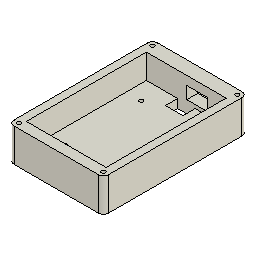
Peekabot 3d design part 1 v1 v21 (Autodesk Fusion 360 design; units mm, degrees)
Autodesk Fusion 360 part; units mm, degrees
sketch "Sketch1" plane through (0, 0, 0) normal (0, 0, 1) x (1, 0, 0)
  line L0 (17.25, -24.75) -> (-17.25, -24.75)
  line L1 (-17.25, -24.75) -> (-17.25, 24.75)
  line L2 (-17.25, 24.75) -> (17.25, 24.75)
  line L3 (17.25, 24.75) -> (17.25, -24.75)
  line L4 (17.25, -24.75) -> (-17.25, 24.75) construction
  line L5 (-17.25, -24.75) -> (17.25, 24.75) construction
  line L6 (-17.25, -24.75) -> (-14.2497, -21.7497)
  line L7 (-17.25, -24.75) -> (-13.007, -24.75) construction
  circle A0 centre (-14.2497, -21.7497) radius 1.115
  line L8 (17.25, -24.75) -> (13.7498, -21.7499)
  line L9 (17.25, -24.75) -> (21.86, -24.75) construction
  circle A1 centre (13.7498, -21.7499) radius 1.115
  line L10 (17.25, 24.75) -> (13.7498, 21.7499)
  line L11 (17.25, 24.75) -> (21.86, 24.75) construction
  circle A2 centre (13.7498, 21.7499) radius 1.1
  line L12 (-17.25, 24.75) -> (-14.2497, 21.7497)
  line L13 (-17.25, 24.75) -> (-13.007, 24.75) construction
  circle A3 centre (-14.2497, 21.7497) radius 1.115
  circle A4 centre (-14.2497, 21.7497) radius 2
  circle A5 centre (13.7498, 21.7499) radius 2
  circle A6 centre (13.7498, -21.7499) radius 2
  circle A7 centre (-14.2497, -21.7497) radius 2
  line L14 (22.25, 29.75) -> (22.25, -29.75)
  line L15 (22.25, -29.75) -> (-22.25, -29.75)
  line L16 (-22.25, -29.75) -> (-22.25, 29.75)
  line L17 (-22.25, 29.75) -> (22.25, 29.75)
  line L18 (27, -41) -> (-27, -41)
  line L19 (-27, -41) -> (-27, 41)
  line L20 (-27, 41) -> (27, 41)
  line L21 (27, 41) -> (27, -41)
  line L22 (27, -41) -> (-27, 41) construction
  line L23 (-27, -41) -> (27, 41) construction
  dimension "d1" = 34.5
  dimension "d2" = 49.5
  dimension "d3" = 45
  dimension "d4" = 4.243
  dimension "d5" = 2.23
  dimension "d6" = 139.4
  dimension "d7" = 4.61
  dimension "d8" = 2.23
  dimension "d9" = 139.4
  dimension "d10" = 4.61
  dimension "d11" = 2.2
  dimension "d12" = 45
  dimension "d13" = 4.243
  dimension "d14" = 2.23
  dimension "d15" = 4
  dimension "d16" = 4
  dimension "d17" = 4
  dimension "d18" = 4
  dimension "d21" = -5
  dimension "d57" = 54
  dimension "d58" = 82
  constraint horizontal L0
  constraint perpendicular L0 L1
  constraint parallel L0 L2
  constraint parallel L1 L3
  constraint coincident L4 origin
  constraint coincident L5 origin
  constraint horizontal L7
  constraint coincident L6.end A0.centre
  constraint horizontal L9
  constraint coincident L8.end A1.centre
  constraint horizontal L11
  constraint coincident L10.end A2.centre
  constraint horizontal L13
  constraint coincident L12.end A3.centre
  constraint concentric A3 A4
  constraint concentric A2 A5
  constraint concentric A1 A6
  constraint concentric A0 A7
  constraint horizontal L18
  constraint perpendicular L18 L19
  constraint parallel L18 L20
  constraint parallel L19 L21
  constraint coincident L22 origin
  constraint coincident L23 origin
  measures "d1" distance of L1.end L2.end
  measures "d2" distance of L0.end L1.end
  measures "d3" angle of L6 L7
  measures "d4" distance of L0.end L6.end
  measures "d5" diameter of A0
  measures "d6" angle of L8 L9
  measures "d7" distance of L0.start L8.end
  measures "d8" diameter of A1
  measures "d9" angle of L10 L11
  measures "d10" distance of L2.end L10.end
  measures "d11" diameter of A2
  measures "d12" angle of L12 L13
  measures "d13" distance of L1.end L12.end
  measures "d14" diameter of A3
  measures "d15" diameter of A4
  measures "d16" diameter of A5
  measures "d17" diameter of A6
  measures "d18" diameter of A7
  measures "d57" distance of L19.end L20.end
  measures "d58" distance of L18.end L19.end
extrude "Extrude1" add sketch "Sketch1" along normal blind 5 contours L0 L1 L2 L3 | A4 | A5 | A6 | A7 makes body 1
extrude "Extrude2" add sketch "Sketch1" along normal blind 5 separate body contours L0 L1 L2 L3 | A4 | A5 | A6 | A7 | L14 L15 L16 L17 makes body 2
extrude "Extrude3" add sketch "Sketch1" along normal blind 19 contours L14 L15 L16 L17 bodies 1 2
extrude "Extrude4" add sketch "Sketch1" against normal blind 5 contours L0 L1 L2 L3 | A6 | A7 | L14 L15 L16 L17 bodies 1
extrude "Extrude5" cut 1 faces at (-17.25, -8.25, 9.6667) along direction (-1, 0, 0) blind 0.5 on bodies 1 bodies 1
extrude "Extrude6" cut 1 faces at (-6.0833, 24.75, 14.3333) along direction (0, 1, 0) blind 0.5 on bodies 1 bodies 1
extrude "Extrude7" cut 1 faces at (17.25, 8.5833, 9.6667) along direction (1, 0, 0) blind 0.5 on bodies 1 bodies 1
extrude "Extrude8" cut 1 faces at (5.9167, -24.75, 9.6667) along direction (0, -1, 0) blind 0.5 on bodies 1 bodies 1
extrude "Extrude9" cut 1 faces at (-5.9167, 25.25, 9.6667) along direction (0, 1, 0) blind 3 on bodies 1 bodies 1
sketch "Sketch2" plane through (0, 29.75, 0) normal (0, 1, 0) x (-1, 0, 0)
  line L0 (22.25, -5) -> (22.25, 19)
  line L1 (22.25, 19) -> (-22.25, 19)
  line L2 (-22.25, 19) -> (-22.25, -5)
  line L3 (-22.25, -5) -> (22.25, -5)
  line L4 (-22.25, 14) -> (-10.25, 14)
  line L5 (-10.25, 14) -> (-0.25, 14)
  line L6 (-0.25, 14) -> (-0.25, 7)
  line L7 (-0.25, 7) -> (-10.25, 7)
  line L8 (-10.25, 7) -> (-10.25, 14)
  line L9 (-22.25, 14) -> (1.75, 14)
  line L10 (1.75, 14) -> (11.75, 14)
  line L11 (11.75, 14) -> (11.75, 7)
  line L12 (11.75, 7) -> (1.75, 7)
  line L13 (1.75, 7) -> (1.75, 14)
  line L14 (-22.25, 19) -> (-22.25, 14)
  dimension "d38" = 12
  dimension "d39" = 10
  dimension "d40" = 7
  dimension "d41" = 24
  dimension "d42" = 10
  dimension "d43" = 7
  dimension "d44" = 5
  constraint coincident L2 L4.start
  constraint perpendicular L2 L4
  constraint horizontal L5
  constraint vertical L6
  constraint horizontal L7
  constraint vertical L8
  constraint perpendicular L6 L9
  constraint horizontal L10
  constraint vertical L11
  constraint horizontal L12
  constraint vertical L13
  constraint coincident L1.end L2.start
  constraint perpendicular L1 L14
  measures "d38" distance of L4.end L4.start
  measures "d39" distance of L4.end L5.end
  measures "d40" distance of L4.end L7.end
  measures "d41" distance of L9.end L4.start
  measures "d42" distance of L9.end L10.end
  measures "d43" distance of L9.end L12.end
  measures "d44" distance of L1.end L4.start
extrude "Extrude10" cut sketch "Sketch2" against normal blind 10 contours L5 L6 L7 L8 L9 | L10 L11 L12 L13 bodies 1
extrude "Extrude11" add 1 faces at (0.25, 29.25, 11.6667) along direction (1, 0, 0) blind 1 on bodies 1 bodies 1
extrude "Extrude12" add sketch "Sketch1" against normal blind 5 contours A5 bodies 1
extrude "Extrude13" add sketch "Sketch1" against normal blind 5 contours A4 bodies 1
extrude "Extrude14" add 1 faces at (0.4167, 29.75, -1) along direction (0, 1, 0) blind 5 on bodies 1 bodies 1
extrude "Extrude15" add sketch "Sketch1" along normal blind 14 separate body contours L18 L19 L20 L21 makes body 3
extrude "Extrude16" add 1 faces at (-7.4167, 37.25, 0) along direction (0, 0, -1) blind 5 on bodies 3 bodies 1 3
extrude "Extrude17" add 1 faces at (7.4167, -37.25, 14) along direction (0, 0, 1) blind 5 on bodies 1 bodies 1
extrude "Extrude18" cut 2 faces at (7.25, 29.75, 11.6667) (-8.4167, 29.75, 11.6667) along direction (0, 1, 0) blind 100 on bodies 1 bodies 1
sketch "Sketch3" plane through (0, 0, -5) normal (0, 0, -1) x (1, 0, 0)
  line L0 (-27, -41) -> (27, -41)
  line L1 (27, -41) -> (27, 41)
  line L2 (27, 41) -> (-27, 41)
  line L3 (-27, 41) -> (-27, -41)
  circle A0 centre (-14.2497, -21.7497) radius 1.115
  circle A1 centre (13.7498, -21.7499) radius 1.1
  circle A2 centre (13.7498, 21.7499) radius 1.115
  circle A3 centre (-14.2497, 21.7497) radius 1.115
  line L4 (27, 41) -> (24.1716, 38.1716)
  line L5 (27, 41) -> (23, 41) construction
  circle A4 centre (24.1716, 38.1716) radius 1.115
  circle A5 centre (24.1716, 38.1716) radius 2
  line L6 (0, 41) -> (0, -41)
  line L7 (27, 0) -> (-27, 0)
  circle A6 centre (-24.1716, 38.1716) radius 1.115
  circle A7 centre (-24.1716, 38.1716) radius 2
  line L8 (-27, 41) -> (-24.1716, 38.1716)
  circle A8 centre (24.1716, -38.1716) radius 2
  circle A9 centre (24.1716, -38.1716) radius 1.115
  line L9 (27, -41) -> (24.1716, -38.1716)
  circle A10 centre (-24.1716, -38.1716) radius 2
  circle A11 centre (-24.1716, -38.1716) radius 1.115
  line L10 (-27, -41) -> (-24.1716, -38.1716)
  dimension "d68" = 45
  dimension "d69" = 4
  dimension "d70" = 2.23
  dimension "d71" = 4
  constraint horizontal L5
  constraint coincident L1.end L2.start
  constraint coincident L4.end A4.centre
  constraint midpoint L2 L6.start
  constraint midpoint L0 L6.end
  constraint midpoint L1 L7.start
  constraint midpoint L3 L7.end
  constraint symmetric L1.end L6 L2.end
  constraint symmetric L4.end L6 A6.centre
  constraint symmetric A4 L6 A6
  constraint symmetric A5 L6 A7
  constraint symmetric L1.end L7 L0.end
  constraint symmetric L4.end L7 A8.centre
  constraint symmetric A4 L7 A9
  constraint symmetric A5 L7 A8
  constraint symmetric L7 A6 A11
  constraint symmetric L7 A7 A10
  constraint symmetric L7 L2.end L0.start
  constraint symmetric L7 A6.centre A10.centre
  measures "d68" angle of L4 L5
  measures "d69" distance of L1.end L4.end
  measures "d70" diameter of A4
  measures "d71" diameter of A5
extrude "Extrude19" cut sketch "Sketch3" against normal blind 15 contours A4 | A6 | A9 | A11 bodies 1
extrude "Extrude20" cut 1 faces at (5.9167, -25.25, 9.6667) along direction (0, -1, 0) blind 10 on bodies 1 bodies 1
extrude "Extrude21" cut 1 faces at (-17.75, -14.0833, 9.6667) along direction (-1, 0, 0) blind 5 on bodies 1 bodies 1
extrude "Extrude22" cut 1 faces at (17.75, 7.0833, 9.6667) along direction (1, 0, 0) blind 5 on bodies 1 bodies 1
extrude "Extrude23" cut 1 faces at (18.5833, 28.25, 12.6667) along direction (0, 1, 0) blind 5 on bodies 1 bodies 1
sketch "Sketch4" plane through (0, 0, 19) normal (0, 0, 1) x (-1, 0, 0)
  line L0 (-27, -41) -> (27, -41)
  line L1 (27, -41) -> (27, 41)
  line L2 (27, 41) -> (-27, 41)
  line L3 (-27, 41) -> (-27, -41)
  line L4 (22.75, 35.25) -> (22.75, -33.25)
  line L5 (22.75, -33.25) -> (-22.75, -33.25)
  line L6 (-22.75, -33.25) -> (-22.75, 35.25)
  line L7 (-22.75, 35.25) -> (22.75, 35.25)
  line L8 (-27, 41) -> (-24.1716, 38.1716)
  line L9 (-27, 41) -> (-23, 41) construction
  circle A0 centre (-24.1716, 38.1716) radius 1.115
  line L10 (0, 41) -> (0, -41)
  line L11 (-27, 0) -> (27, 0)
  circle A1 centre (24.1716, 38.1716) radius 1.115
  circle A2 centre (-24.1716, -38.1716) radius 1.115
  circle A3 centre (24.1716, -38.1716) radius 1.115
  dimension "d82" = 45
  dimension "d83" = 4
  dimension "d84" = 2.23
  constraint horizontal L9
  constraint coincident L2.end L3.start
  constraint coincident L8.end A0.centre
  constraint midpoint L2 L10.start
  constraint midpoint L0 L10.end
  constraint midpoint L3 L11.start
  constraint midpoint L1 L11.end
  constraint symmetric A0 L10 A1
  constraint symmetric A0 L11 A2
  constraint symmetric L11 A1 A3
  measures "d82" angle of L8 L9
  measures "d83" distance of L2.end L8.end
  measures "d84" diameter of A0
extrude "Extrude24" cut sketch "Sketch4" against normal blind 10 contours A0 | A1 | A2 | A3 bodies 1
extrude "Extrude25" cut 1 faces at (4.2333, 6.9324, -5) along direction (0, 0, 1) blind 5 on bodies 1 bodies 1
fillet "Fillet1" radius 4 4 edges at (27, -41, 9.5) (-27, -41, 9.5) (27, 41, 9.5) (-27, 41, 9.5) on bodies 1
sketch "Sketch6" plane through (0, 0, 5) normal (0, 0, 1) x (-1, 0, 0)
  line L0 (22.75, -33.25) -> (22.75, 35.25)
  line L1 (22.75, 35.25) -> (-22.75, 35.25)
  line L2 (-22.75, 35.25) -> (-22.75, -33.25)
  line L3 (-22.75, -33.25) -> (22.75, -33.25)
  circle A0 centre (14.2497, -21.7497) radius 1.115
  circle A1 centre (-13.7498, 21.7499) radius 1.115
  circle A2 centre (-13.7498, -21.7499) radius 1.1
  circle A3 centre (14.2497, 21.7497) radius 1.115
  line L4 (-5.067, -33.25) -> (4.933, -33.25)
  line L5 (4.933, -33.25) -> (4.933, -26.25)
  line L6 (4.933, -26.25) -> (-5.067, -26.25)
  line L7 (-5.067, -26.25) -> (-5.067, -33.25)
  dimension "d105" = 10
  dimension "d106" = 7
  constraint horizontal L4
  constraint vertical L5
  constraint horizontal L6
  constraint vertical L7
  constraint coincident L3 L4.start
  measures "d105" distance of L4.start L4.end
  measures "d106" distance of L4.start L6.end
extrude "Extrude31" cut sketch "Sketch6" against normal blind 100 contours L3 L4 L5 L6 L7 bodies 1
extrude "Extrude32" add 1 faces at (-5.0833, 38.4167, 7) along direction (0, 0, 1) blind 7 on bodies 1 bodies 1
extrude "Extrude33" cut 1 faces at (1.25, 38.4167, 9.3333) along direction (-1, 0, 0) blind 1.5 on bodies 1 bodies 1
extrude "Extrude34" cut 1 faces at (10.25, 35.8333, 9.3333) along direction (1, 0, 0) blind 1.5 on bodies 1 bodies 1
extrude "Extrude35" cut 1 faces at (11.75, 35.8333, 9.3333) along direction (1, 0, 0) blind 1 on bodies 1 bodies 1
extrude "Extrude36" add 1 faces at (-0.25, 38.4167, 9.3333) along direction (1, 0, 0) blind 1 on bodies 1 bodies 1
extrude "Extrude37" add 1 faces at (12.75, 35.8333, 9.3333) along direction (-1, 0, 0) blind 0.5 on bodies 1 bodies 1
extrude "Extrude38" cut 1 faces at (0.75, 38.4167, 9.3333) along direction (-1, 0, 0) blind 0.5 on bodies 1 bodies 1
fillet "Fillet4" radius 1.5 4 edges at (0.25, 41, 10.5) (6.25, 41, 14) (6.25, 41, 7) (12.25, 41, 10.5) on bodies 1
delete_face "DeleteFace1" 1 faces at (26.9955, -37.1903, 6.3333) on bodies 1
delete_face "DeleteFace2" 1 faces at (23.1903, 40.9955, 6.3333) on bodies 1
delete_face "DeleteFace3" 1 faces at (-23.1903, 40.9955, 12.6667) on bodies 1
delete_face "DeleteFace4" 1 faces at (-26.9955, -37.1903, 12.6667) on bodies 1
fillet "Fillet5" radius 3 4 edges at (27, -41, 9.5) (27, 41, 9.5) (-27, -41, 9.5) (-27, 41, 9.5) on bodies 1
extrude "Extrude26" [suppressed]
extrude "Extrude27" [suppressed]
extrude "Extrude28" [suppressed]
extrude "Extrude29" [suppressed]
sketch "Sketch5" plane through (0, 0, 0) normal (0, 0, -1) x (1, 0, 0)
  arc A0 (-27, -37) -> (-23, -41) centre (-23, -37) ccw
  line L0 (-23, -41) -> (-23, -42)
  line L1 (-23, -42) -> (23, -42)
  line L2 (23, -42) -> (23, -41)
  arc A1 (23, -41) -> (27, -37) centre (23, -37) ccw
  line L3 (27, -37) -> (28, -37)
  line L4 (28, -37) -> (28, 37)
  line L5 (28, 37) -> (27, 37)
  arc A2 (27, 37) -> (23, 41) centre (23, 37) ccw
  line L6 (23, 41) -> (23, 42)
  line L7 (23, 42) -> (-23, 42)
  line L8 (-23, 42) -> (-23, 41)
  arc A3 (-23, 41) -> (-27, 37) centre (-23, 37) ccw
  line L9 (-27, 37) -> (-28, 37)
  line L10 (-28, 37) -> (-28, -37)
  line L11 (-28, -37) -> (-27, -37)
  circle A4 centre (-14.2497, 21.7497) radius 1.115
  circle A5 centre (13.7498, 21.7499) radius 1.115
  circle A6 centre (13.7498, -21.7499) radius 1.1
  circle A7 centre (-14.2497, -21.7497) radius 1.115
  circle A8 centre (-24.1716, -38.1716) radius 1.115
  circle A9 centre (24.1716, 38.1716) radius 1.115
  circle A10 centre (-24.1716, 38.1716) radius 1.115
  circle A11 centre (24.1716, -38.1716) radius 1.115
  line L12 (28, -42) -> (-28, -42)
  line L13 (-28, -42) -> (-28, 42)
  line L14 (-28, 42) -> (28, 42)
  line L15 (28, 42) -> (28, -42)
  constraint horizontal L12
  constraint vertical L13
  constraint horizontal L14
  constraint vertical L15
extrude "Extrude30" [suppressed]
fillet "Fillet2" [suppressed]
fillet "Fillet3" [suppressed]
equation "d24 = 5 mm + 14 mm"
